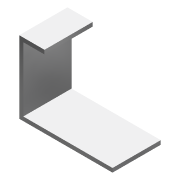
# Autodesk Inventor part: body_2
Saved by Autodesk Inventor 2014 (Build 180170000, 170)
## iProperties
Created: 2015-11-19
Part Number: body_2
Material: Generic
Document SubType Name: Modeling
Designer: Tom
Density: 1 g/cm^3
Appearance: Default
Author: Tom
Autodesk Inventor part; units mm, degrees
ref_plane "YZ Plane" through (0, 0, 0) normal (1, 0, 0) x (0, 1, 0)
ref_plane "XZ Plane" through (0, 0, 0) normal (0, 1, 0) x (-1, 0, 0)
ref_plane "XY Plane" through (0, 0, 0) normal (0, 0, 1) x (1, 0, 0)
sketch "Sketch1" plane through (0, 0, 0) normal (0, 0, 1) x (1, 0, 0)
  line L0 (-1.3413, -0.4194) -> (0, -0.4194)
  line L1 (-1.3413, -4.7374) -> (-1.3413, -0.4194)
  line L2 (0, -0.1654) -> (-1.5953, -0.1654)
  line L3 (-1.5953, -0.1654) -> (-1.5953, -4.7374)
  line L4 (-1.3413, -4.7374) -> (-1.5953, -4.7374)
  line L5 (0, -0.4194) -> (0, -0.1654)
  point P0 (0, 0)
  dimension "d1" = 0.254
  dimension "d8" = 4.572
  constraints: 12 end point, 2 perpendicular, 1 horizontal, 1 other
  measures "d1" distance between parallel lines of L2 L0
  measures "d8" distance of L2.end L3.end
extrude "Extrusion1" add sketch "Sketch1" along normal blind 3.048
sketch "Sketch2" plane through (0, 0, 3.048) normal (0, 0, 1) x (1, 0, 0)
  line L0 (-1.3413, -4.7374) -> (4.2975, -4.7374)
  line L1 (4.2975, -4.7374) -> (4.2975, -4.4834)
  line L2 (4.2975, -4.4834) -> (-1.3413, -4.4834)
  line L3 (-1.3413, -4.4834) -> (-1.3413, -4.7374)
  dimension "d4" = 5.6388
  dimension "d5" = 0.254
  constraints: 8 end point, 2 parallel, 1 horizontal, 1 perpendicular
  measures "d4" distance of L2.end L1.end
  measures "d5" distance of L1.end L0.end
extrude "Extrusion2" add sketch "Sketch2" against normal up to surface (3.048 mm away)
body "Solid1"
